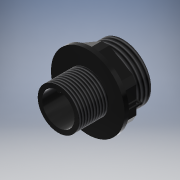
# Autodesk Inventor part: nut
Saved by Autodesk Inventor 2018 (Build 220112000, 112)
## iProperties
Created: 2019-04-16
Part Number: nut
Material: Generic
Document SubType Name: Modeling
Designer: ZEUSLAP
Density: 1 g/cm^3
Appearance: Default
Author: ZEUSLAP
Autodesk Inventor part; units mm, degrees
ref_plane "YZ Plane" through (0, 0, 0) normal (1, 0, 0) x (0, 1, 0)
ref_plane "XZ Plane" through (0, 0, 0) normal (0, 1, 0) x (-1, 0, 0)
ref_plane "XY Plane" through (0, 0, 0) normal (0, 0, 1) x (1, 0, 0)
sketch "Sketch1" plane through (0, 0, 0) normal (0, 1, 0) x (-1, 0, 0)
  circle A0 centre (0, 0) radius 5.5
  circle A1 centre (0, 0) radius 7
  dimension "d0" = 11
  dimension "d1" = 14
  constraints: 2 centre point, 2 coincident
  measures "d0" diameter of A0
  measures "d1" diameter of A1
extrude "Extrusion1" add sketch "Sketch1" along normal blind 10
thread "Thread1" size "M14x1" class "6g" standard "ANSI Metric M Profile" full length
sketch "Sketch2" plane through (0, 0, 0) normal (0, -1, 0) x (1, 0, 0)
  circle A0 centre (0, 5.4798) radius 0.75
  point P0 (0, 0)
  dimension "d6" = 1.5
  constraints: 1 centre point
  measures "d6" diameter of A0
extrude "Extrusion2" add sketch "Sketch2" against normal blind 10
sketch "Sketch3" plane through (0, 10, 0) normal (0, 1, 0) x (1, 0, 0)
  circle A0 centre (0, 0) radius 5.5
  circle A1 centre (0, 0) radius 12.5
  dimension "d9" = 11
  dimension "d10" = 25
  constraints: 2 centre point, 2 coincident
  measures "d9" diameter of A0
  measures "d10" diameter of A1
extrude "Extrusion3" add sketch "Sketch3" along normal blind 1.5 contours A0 | A1
sketch "Sketch4" plane through (0, 11.5, 0) normal (0, 1, 0) x (1, 0, 0)
  line L0 (10.5, -6.0622) -> (0, -12.1244)
  line L1 (0, -12.1244) -> (-10.5, -6.0622)
  line L2 (-10.5, -6.0622) -> (-10.5, 6.0622)
  line L3 (-10.5, 6.0622) -> (0, 12.1244)
  line L4 (0, 12.1244) -> (10.5, 6.0622)
  line L5 (10.5, 6.0622) -> (10.5, -6.0622)
  circle A0 centre (0, 0) radius 7.5
  dimension "d14" = 15
  constraints: 12 end point, 2 coincident, 1 centre point, 1 other
  measures "d14" diameter of A0
extrude "Extrusion4" add sketch "Sketch4" along normal blind 4.5
sketch "Sketch5" plane through (0, 16, 0) normal (0, 1, 0) x (1, 0, 0)
  circle A0 centre (0, 0) radius 7.5
  circle A1 centre (0, 0) radius 9.5
  dimension "d17" = 15
  dimension "d18" = 19
  constraints: 2 centre point, 2 coincident
  measures "d17" diameter of A0
  measures "d18" diameter of A1
extrude "Extrusion5" add sketch "Sketch5" along normal blind 6
thread "Thread2" size "M20x1.5" class "6g" standard "ANSI Metric M Profile" full length
sketch "Sketch6" plane through (0, 22, 0) normal (0, 1, 0) x (1, 0, 0)
  line L0 (0.5, -8.4949) -> (-0.5, -8.4949)
  line L1 (-0.5, -8.4949) -> (-0.5, -6.4949)
  line L2 (-0.5, -6.4949) -> (0.5, -6.4949)
  line L3 (0.5, -6.4949) -> (0.5, -8.4949)
  line L4 (0.5, -8.4949) -> (-0.5, -6.4949) construction
  line L5 (-0.5, -8.4949) -> (0.5, -6.4949) construction
  line L6 (3.8144, 7.6068) -> (4.6804, 7.1068)
  line L7 (4.6804, 7.1068) -> (3.6804, 5.3747)
  line L8 (3.6804, 5.3747) -> (2.8144, 5.8747)
  line L9 (2.8144, 5.8747) -> (3.8144, 7.6068)
  line L10 (3.8144, 7.6068) -> (3.6804, 5.3747) construction
  line L11 (4.6804, 7.1068) -> (2.8144, 5.8747) construction
  line L12 (-4.6804, 7.1068) -> (-3.8144, 7.6068)
  line L13 (-3.8144, 7.6068) -> (-2.8144, 5.8747)
  line L14 (-2.8144, 5.8747) -> (-3.6804, 5.3747)
  line L15 (-3.6804, 5.3747) -> (-4.6804, 7.1068)
  line L16 (-4.6804, 7.1068) -> (-2.8144, 5.8747) construction
  line L17 (-3.8144, 7.6068) -> (-3.6804, 5.3747) construction
  point P0 (0, 0)
  point P1 (0, -7.4949)
  point P2 (0, 0)
  point P3 (3.7474, 6.4907)
  point P4 (-3.7474, 6.4907)
  dimension "d23" = 1
  dimension "d24" = 2
  dimension "d27" = 150
  dimension "d31" = 210
  constraints: 36 end point, 6 midpoint, 2 parallel, 1 coincident, 1 horizontal, 1 perpendicular, 24 other
  measures "d23" distance of L1.end L2.end
  measures "d24" distance of L0.end L1.end
extrude "Extrusion6" add sketch "Sketch6" against normal blind 10.5
chamfer "Chamfer1" distance 1.5 angle 45 6 edges at (-10.5, 13.75, 6.0622) (-10.5, 13.75, -6.0622) (0, 13.75, 12.1244) (10.5, 13.75, 6.0622) (10.5, 13.75, -6.0622) (0, 13.75, -12.1244)
sketch "Sketch8" plane through (0, 0, 0) normal (0, 0, 1) x (1, 0, 0)
  line L0 (10.5, 16) -> (9.201, 16) projected
  line L1 (12.5, 11.5) -> (-12.5, 11.5) projected
  line L2 (10.5, 16) -> (12.5, 16)
  line L3 (12.5, 16) -> (12.5, 11.5)
  line L4 (12.5, 11.5) -> (10.5, 11.5)
  line L5 (10.5, 11.5) -> (10.5, 16)
  line L6 (-10.5, 16) -> (-10.5, 11.5) projected
  line L7 (-12.5, 11.5) -> (-10.5, 11.5)
  line L8 (-10.5, 11.5) -> (-10.5, 16)
  line L9 (-10.5, 16) -> (-12.5, 16)
  line L10 (-12.5, 16) -> (-12.5, 11.5)
  line L11 (-13, 11) -> (-10, 11)
  line L12 (-10, 11) -> (-10, 16.5)
  line L13 (-10, 16.5) -> (-13, 16.5)
  line L14 (-13, 16.5) -> (-13, 11)
  line L15 (12, 12) -> (12, 15.5)
  line L16 (12, 15.5) -> (11, 15.5)
  line L17 (11, 15.5) -> (11, 12)
  line L18 (11, 12) -> (12, 12)
  dimension "d43" = 0.5
  dimension "d44" = 0.5
  constraints: 32 end point, 8 parallel, 4 perpendicular, 2 horizontal, 6 other
  measures "d43" distance between parallel lines of L10 L14
  measures "d44" distance between parallel lines of L3 L15
extrude "Extrusion8" add sketch "Sketch8" along normal mid plane 0.5
body "Solid1"
